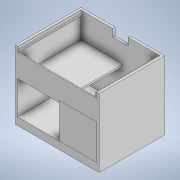
# Autodesk Inventor part: circuit casing
Saved by Autodesk Inventor 2022 (Build 260153000, 153)
## iProperties
Created: 2023-02-06
Part Number: circuit casing
Material: Generic
Document SubType Name: Modeling
Designer: biom
Density: 1 g/cm^3
Appearance: Default
Author: biom
Autodesk Inventor part; units mm, degrees
ref_plane "YZ Plane" through (0, 0, 0) normal (1, 0, 0) x (0, 1, 0)
ref_plane "XZ Plane" through (0, 0, 0) normal (0, 1, 0) x (-1, 0, 0)
ref_plane "XY Plane" through (0, 0, 0) normal (0, 0, 1) x (1, 0, 0)
sketch "Sketch12" plane through (0, 0, 0) normal (0, 1, 0) x (-1, 0, 0)
  line L0 (0, 0) -> (110, 0)
  line L1 (110, 0) -> (110, -86)
  line L2 (110, -86) -> (0, -86)
  line L3 (0, -86) -> (0, 0)
  dimension "d23" = 110
  dimension "d24" = 86
  constraints: 8 end point, 2 parallel, 1 horizontal, 1 perpendicular
  measures "d23" distance of L1.end L2.end
  measures "d24" distance of L0.end L1.end
extrude "Extrusion6" add sketch "Sketch12" along normal blind 10
sketch "Sketch13" plane through (0, 10, 0) normal (0, 1, 0) x (1, 0, 0)
  line L0 (0, 0) -> (0, 86) projected
  line L1 (-110, 0) -> (0, 0) projected
  line L2 (0, 86) -> (-110, 86) projected
  line L3 (-110, 86) -> (-110, 0) projected
  line L4 (-107, 43) -> (-107, 83)
  line L5 (-107, 83) -> (-107, 0)
  line L6 (-107, 83) -> (-3, 83)
  line L7 (-3, 0) -> (-3, 83)
  constraints: 8 end point, 2 point on line, 1 perpendicular
extrude "Extrusion7" add sketch "Sketch13" along normal blind 80 contours L1 L7 L6 L4 L5 L3 L2 L0
sketch "Sketch14" plane through (-107, 10, -83) normal (0, 0, 1) x (1, 0, 0)
  line L0 (0, 80) -> (104, 80) projected
  line L1 (62, 80) -> (42, 80)
  line L2 (42, 80) -> (42, 70)
  line L3 (42, 70) -> (62, 70)
  line L4 (62, 70) -> (62, 80)
  point P0 (107, -10)
  dimension "d33" = 20
  dimension "d34" = 10
  dimension "d35" = 20
  constraints: 8 end point, 1 perpendicular, 1 point on line, 1 vertical
  measures "d33" distance of L1.start L1.end
  measures "d34" distance of L1.end L2.end
  measures "d35" distance of L2.end L3.end
extrude "Extrusion8" cut sketch "Sketch14" against normal through all
sketch "Sketch15" plane through (-107, 10, 0) normal (1, 0, 0) x (0, 0, -1)
  line L0 (0, 80) -> (83, 80) projected
  line L1 (41.5, 79) -> (83, 79)
  line L2 (83, 0) -> (83, 80) projected
  line L3 (83, 79) -> (0, 79)
  line L4 (0, 0) -> (0, 80) projected
  line L5 (0, 79) -> (0, 77.5)
  line L6 (0, 77.5) -> (83, 77.5)
  line L7 (0, 76) -> (83, 76)
  line L8 (83, 76) -> (83, 74.5)
  line L9 (83, 74.5) -> (0, 74.5)
  line L10 (0, 76) -> (0, 74.5)
  line L11 (83, 79) -> (83, 77.5)
  point P0 (0, -10)
  dimension "d39" = 1.5
  dimension "d40" = 1.5
  dimension "d41" = 1.5
  constraints: 18 end point, 7 point on line, 4 perpendicular, 2 collinear
  measures "d39" distance of L3.end L5.end
  measures "d40" distance of L5.end L7.start
  measures "d41" distance of L7.end L8.end
extrude "Extrusion9" add sketch "Sketch15" along normal blind 2 contours L3 L1 L2 L6 L4 | L7 L2 L9 L4
sketch "Sketch16" plane through (-3, 10, -83) normal (-1, 0, 0) x (0, 0, 1)
  line L0 (0, 80) -> (83, 80) projected
  line L1 (41.5, 79) -> (0, 79)
  line L2 (0, 0) -> (0, 80) projected
  line L3 (0, 79) -> (83, 79)
  line L4 (83, 0) -> (83, 80) projected
  line L5 (83, 79) -> (83, 77.5)
  line L6 (83, -10) -> (83, 80) projected
  line L7 (83, 77.5) -> (0, 77.5)
  line L8 (0, 77.5) -> (0, 79)
  line L9 (0, 76) -> (83, 76)
  line L10 (83, 76) -> (83, 74.5)
  line L11 (83, 74.5) -> (0, 74.5)
  line L12 (0, 74.5) -> (0, 76)
  point P0 (0, 74.5)
  point P1 (0, 76)
  dimension "d45" = 1.5
  dimension "d46" = 1.5
  dimension "d47" = 1.5
  constraints: 18 end point, 7 point on line, 4 perpendicular, 1 parallel
  measures "d45" distance of L3.end L5.end
  measures "d46" distance of L7.end L9.start
  measures "d47" distance of L9.end L10.end
extrude "Extrusion10" add sketch "Sketch16" along normal blind 2 contours L1 L3 L4 L7 L2 | L9 L4 L11 L2
sketch "Sketch17" plane through (-107, 10, 0) normal (1, 0, 0) x (0, 0, -1)
  line L0 (83, 74.5) -> (0, 74.5) projected
  line L1 (0, 0) -> (0, 74.5) projected
  line L2 (0, 43.5) -> (83, 43.5)
  line L3 (83, 0) -> (83, 74.5) projected
  line L4 (83, 43.5) -> (83, 46)
  line L5 (83, 46) -> (0, 45.9998)
  line L6 (0, 45.9998) -> (0, 43.5)
  point P0 (0, -10)
  dimension "d50" = 31
  dimension "d51" = 2.5
  constraints: 8 end point, 4 point on line, 1 perpendicular
  measures "d50" distance of L0.end L2.start
  measures "d51" distance of L2.end L4.end
extrude "Extrusion11" add sketch "Sketch17" along normal blind 55 contours L3 L2 L1 L5
sketch "Sketch18" plane through (-107, 84.5, 0) normal (1, 0, 0) x (0, 0, -1)
  line L0 (0, -84.5) -> (0, 5.5) projected
  line L1 (0, -28.5002) -> (0, 0) projected
  line L2 (0, -1.5292) -> (0, -28.5002)
  line L3 (0, -28.5002) -> (1.25, -28.5002)
  line L4 (0, -28.5002) -> (83, -28.5) projected
  line L5 (1.25, -28.5002) -> (1.25, -1.5292)
  line L6 (1.25, -1.5292) -> (0, -1.5292)
  dimension "d54" = 1.25
  dimension "d55" = 26.971
  constraints: 8 end point, 2 point on line, 1 collinear, 1 perpendicular, 1 vertical
  measures "d54" distance of L1.start L3.end
  measures "d55" distance of L3.end L5.end
extrude "Extrusion12" add sketch "Sketch18" along normal up to surface (104 mm away)
sketch "Sketch19" plane through (-52, 55.9998, -1.25) normal (0, -1, 0) x (1, 0, 0)
  line L0 (0, 0) -> (0, 1.25) projected
  line L1 (0, 1.25) -> (49, 1.25) projected
  line L2 (0, 1.25) -> (49, 1.25)
  line L3 (49, 1.25) -> (49, 0) projected
  line L4 (49, 1.25) -> (49, 0)
  line L5 (0, 0) -> (49, 0) projected
  line L6 (0, 1.25) -> (0, 0)
  line L7 (0, -81.75) -> (0, 0) projected
  line L8 (0, 0) -> (49, 0)
  point P0 (52, 1.2502)
  constraints: 8 end point, 2 collinear, 1 horizontal, 1 perpendicular
extrude "Extrusion13" add sketch "Sketch19" along normal up to surface (45.9998 mm away)
sketch "Sketch20" plane through (-110, 0, 0) normal (0, 0, 1) x (1, 0, 0)
  point P0 (110, 0)
body "Solid3"
